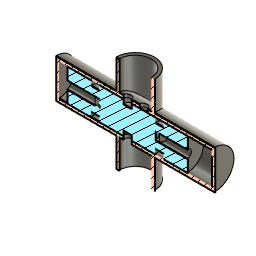
Timer v4 (Autodesk Fusion 360 design; units mm, degrees)
Autodesk Fusion 360 part; units mm, degrees
sketch "Piston" plane through (0, 0, 0) normal (0, 1, 0) x (1, 0, 0)
  line L0 (0, -10) -> (15, -10)
  line L1 (15, -10) -> (15, -7)
  line L2 (15, -7) -> (20, -7)
  line L3 (20, -7) -> (20, -10)
  line L4 (20, -10) -> (35, -10)
  line L5 (35, -10) -> (35, -7)
  line L6 (35, -7) -> (40, -7)
  line L7 (40, -7) -> (40, -10)
  line L8 (40, -10) -> (55, -10)
  line L9 (55, -10) -> (55, -7)
  line L10 (55, -7) -> (60, -7)
  line L11 (60, -7) -> (60, -10)
  line L12 (60, -10) -> (75, -10)
  line L13 (75, -10) -> (75, 0)
  line L14 (75, 0) -> (0, 0)
  line L15 (0, 0) -> (0, -10)
  line L16 (0, -2.5) -> (20, -2.5)
  line L17 (20, -2.5) -> (20, 0)
  line L18 (75, -2.5) -> (55, -2.5)
  line L19 (55, -2.5) -> (55, 0)
  dimension "d1" = 5
  dimension "d2" = 5
  dimension "d3" = 5
  dimension "d4" = 15
  dimension "d5" = 15
  dimension "d6" = 15
  dimension "d7" = 15
  dimension "d8" = 10
  dimension "d9" = 7
  dimension "d10" = 10
  dimension "d11" = 7
  dimension "d12" = 10
  dimension "d13" = 7
  dimension "d14" = 10
  dimension "d15" = 2.5
  dimension "d16" = 20
  dimension "d17" = 2.5
  dimension "d18" = 20
  constraint horizontal L0
  constraint perpendicular L0 L1
  constraint perpendicular L1 L2
  constraint perpendicular L0 L3
  constraint perpendicular L3 L4
  constraint perpendicular L4 L5
  constraint perpendicular L5 L6
  constraint perpendicular L6 L7
  constraint perpendicular L7 L8
  constraint perpendicular L6 L9
  constraint perpendicular L7 L10
  constraint perpendicular L10 L11
  constraint perpendicular L11 L12
  constraint perpendicular L12 L13
  constraint coincident L14.end L15.start
  constraint perpendicular L13 L14
  constraint perpendicular L0 L15
  constraint coincident L15 L16.start
  constraint perpendicular L15 L16
  constraint coincident L14 L17.end
  constraint perpendicular L14 L17
  constraint coincident L13 L18.start
  constraint perpendicular L13 L18
  constraint coincident L14 L19.end
  constraint perpendicular L14 L19
  measures "d1" distance of L1.end L2.end
  measures "d2" distance of L5.end L6.end
  measures "d3" distance of L9.end L10.end
  measures "d4" distance of L11.end L12.end
  measures "d5" distance of L7.end L8.end
  measures "d6" distance of L3.end L4.end
  measures "d7" distance of L0.start L0.end
  measures "d8" distance of L0.start L14.end
  measures "d9" distance of L2 L14
  measures "d10" distance of L4 L14
  measures "d11" distance of L6 L14
  measures "d12" distance of L8 L14
  measures "d13" distance of L10 L14
  measures "d14" distance of L12 L14
  measures "d15" distance of L14 L16
  measures "d16" distance of L16.start L16.end
  measures "d17" distance of L14 L18
  measures "d18" distance of L13 L19
sketch "Cylinder" plane through (0, 0, 0) normal (0, 1, 0) x (1, 0, 0)
  line L0 (-5, 0) -> (-5, -10)
  line L1 (-5, -10) -> (90, -10)
  line L2 (90, -10) -> (90, 0)
  line L3 (90, 0) -> (92, 0)
  line L4 (92, 0) -> (92, -12)
  line L5 (92, -12) -> (-7, -12)
  line L6 (-7, -12) -> (-7, 0)
  line L7 (-7, 0) -> (-5, 0)
  line L8 (75, -10) -> (75, 0)
  line L9 (0, 0) -> (0, -10)
  line L10 (15, -7) -> (20, -7)
  line L11 (35, -7) -> (40, -7)
  line L12 (55, -7) -> (60, -7)
  circle A0 centre (17.5, 0.008) radius 2.5
  circle A1 centre (37.5, 0) radius 2.5
  circle A2 centre (57.5, -0.0105) radius 2.5
  circle A3 centre (47.5, 0) radius 2.5
  circle A4 centre (37.5, 0) radius 2.5
  circle A5 centre (27.5, 0) radius 2.5
  circle A6 centre (67.5, 0) radius 2.5
  circle A7 centre (17.5, 0.008) radius 4.5
  circle A8 centre (67.5, 0) radius 4.5
  dimension "d20" = 2
  dimension "d21" = 2
  dimension "d22" = 2
  dimension "d24" = 5
  dimension "d25" = 15
  dimension "d26" = 5
  dimension "d27" = 5
  dimension "d28" = 5
  dimension "d29" = 5
  dimension "d30" = 5
  dimension "d31" = 5
  dimension "d32" = 5
  dimension "d40" = 2
  dimension "d41" = 2
  constraint vertical L0
  constraint perpendicular L0 L1
  constraint perpendicular L1 L2
  constraint perpendicular L0 L3
  constraint perpendicular L3 L4
  constraint perpendicular L4 L5
  constraint perpendicular L5 L6
  constraint perpendicular L0 L7
  measures "d20" distance of L0 L6
  measures "d21" distance of L1 L5
  measures "d22" distance of L2 L4
  measures "d24" distance of L0 L9
  measures "d25" distance of L2 L8
  measures "d26" diameter of A0
  measures "d27" diameter of A1
  measures "d28" diameter of A2
  measures "d29" diameter of A3
  measures "d30" diameter of A4
  measures "d31" diameter of A5
  measures "d32" diameter of A6
sketch "In/out ports" plane through (0, 0, 0) normal (0, 0, 1) x (1, 0, 0)
  circle A0 centre (42.5, 0) radius 10
  circle A1 centre (37.5, 0) radius 2.5
  circle A2 centre (47.5, 0) radius 2.5
  circle A3 centre (42.5, 0) radius 12
  point P0 (47.5, 0)
  point P1 (37.5, 0)
  dimension "d52" = 20
  dimension "d53" = 5
  dimension "d54" = 5
  dimension "d55" = 5
  dimension "d56" = 24
  constraint coincident P1 A1.centre
  constraint coincident P0 A2.centre
  constraint concentric A0 A3
  measures "d52" diameter of A0
  measures "d53" distance of P1 A0.centre
  measures "d54" diameter of A1
  measures "d55" diameter of A2
  measures "d56" diameter of A3
revolve "Revolve2" add sketch "Cylinder" angle 360 about axis through (1.75, 0, 0) along (1, 0, 0) contours L0 L1 L2 L3 L4 L5 L6 L7 makes body 1
extrude "Extrude10" add sketch "In/out ports" along normal mid plane 60 contours A3 bodies 1
extrude "Extrude11" cut 1 faces at (90, -1.6624, 3.4521) along direction (-1, 0, 0) up to surface (95 mm away) on bodies 1 bodies 1
extrude "Extrude12" cut sketch "In/out ports" along normal through all and the other way through all contours A1 bodies 1
extrude "Extrude13" cut sketch "In/out ports" along normal through all contours A2 bodies 1
revolve "Revolve1" add sketch "Piston" angle 360 about axis through (75, 0, 0) along (-1, 0, 0) separate body contours L0 L1 L2 L3 L4 L5 L6 L7 L8 L9 L10 L11 L12 L13 L14 L15 L16 L17 L18 L19 makes body 2
extrude "Extrude1" cut sketch "Cylinder" along normal through all and the other way through all contours A0 | A2 bodies 2
extrude "Extrude2" cut sketch "Cylinder" along normal through all contours A2 | A3 | A5 bodies 1
sketch "Side tube" plane through (-7, 0, 0) normal (-1, 0, 0) x (0, -1, 0)
  circle A0 centre (0, 0) radius 12
  circle A1 centre (16.5, 0) radius 4.5
  circle A2 centre (16.5, 0) radius 2.5
  dimension "d36" = 9
  dimension "d37" = 5
  constraint concentric A1 A2
  measures "d36" diameter of A1
  measures "d37" diameter of A2
extrude "Extrude3" add sketch "Side tube" against normal up to surface (99 mm away) separate body contours A1 makes body 3
extrude "Extrude4" cut sketch "Cylinder" against normal blind 16.5 contours A0 | A6 bodies 1 3
extrude "Extrude6" add sketch "Cylinder" against normal blind 6.5 from surface at -10 separate body contours A7 | A8 makes body 4 at (68.7188, -14.3333, -4.3318) makes body 5 at (21.9776, -12.1667, 0.4401)
extrude "Extrude7" cut sketch "Side tube" against normal through all contours A2 bodies 4 5
combine "Combine1" operation add target body 3 tool bodies 4 5
extrude "Extrude14" add sketch "Side tube" against normal blind 2 contours A2 bodies 3
combine "Combine2" operation add target body 1 tool bodies 3
copy_body "Body->Comp1" bodies 1 removing the originals makes body 6 in component "Cylinder"
copy_body "Body->Comp2" bodies 2 removing the originals makes body 7 in component "Piston"
component "Cylinder" placed x (1, 0, 0) y (0, 1, 0) z (0, 0, 1) at (0, 0, 0)
component "Piston" placed x (1, 0, 0) y (0, 1, 0) z (0, 0, 1) at (0, 0, 0)
equation "d10 = d8"
equation "d11 = d9"
equation "d12 = d10"
equation "d13 = d11"
equation "d14 = d8"
equation "d17 = d15"
equation "d18 = d16"
equation "d21 = d20"
equation "d22 = d20"
named bodies: "Piston", "Cylinder"
